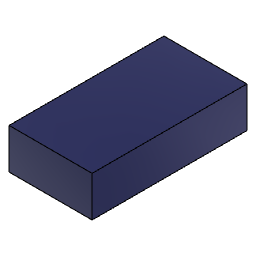
Onboard Gateway (FINAL) v33 (Autodesk Fusion 360 archive; units mm, degrees)
design "4400 mAh"
Autodesk Fusion 360 part; units mm, degrees
sketch "Sketch1" plane through (0, 0, 0) normal (0, 0, 1) x (1, 0, 0)
  line L0 (-19.6609, 33.9067) -> (17.3391, 33.9067)
  line L1 (17.3391, 33.9067) -> (17.3391, -35.0933)
  line L2 (17.3391, -35.0933) -> (-19.6609, -35.0933)
  line L3 (-19.6609, -35.0933) -> (-19.6609, 33.9067)
  dimension "d1" = 69
  dimension "d2" = 37
  constraint horizontal L0
  constraint vertical L1
  constraint horizontal L2
  constraint vertical L3
  measures "d1" distance of L0.start L2.end
  measures "d2" distance of L0.start L0.end
extrude "Extrude1" add sketch "Sketch1" along normal blind 18

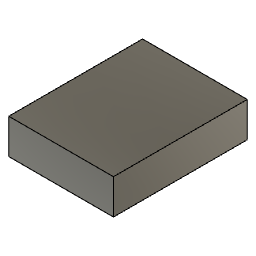
design "6600 mAh"
Autodesk Fusion 360 part; units mm, degrees
sketch "Sketch1" plane through (0, 0, 0) normal (0, 0, 1) x (1, 0, 0)
  line L0 (-27.2206, 35.9271) -> (26.7794, 35.9271)
  line L1 (26.7794, 35.9271) -> (26.7794, -33.0729)
  line L2 (26.7794, -33.0729) -> (-27.2206, -33.0729)
  line L3 (-27.2206, -33.0729) -> (-27.2206, 35.9271)
  dimension "d1" = 69
  dimension "d2" = 54
  constraint horizontal L0
  constraint vertical L1
  constraint horizontal L2
  constraint vertical L3
  measures "d1" distance of L0.start L2.end
  measures "d2" distance of L0.start L0.end
extrude "Extrude1" add sketch "Sketch1" along normal blind 18
